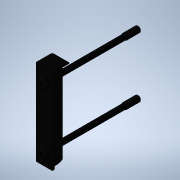
# Autodesk Inventor part: 8092760 MS4-MV-B---(46_high_m)
Saved by Autodesk Inventor 2024.3 (Build 283343000, 343)
## iProperties
Category: PARTsolutions
Company: FESTO
Created: 2025-04-26
Part Number: 8092760 MS4-MV-B---(46_high_m)
Material: Generic
Catalog Web Link: www.cadenas.de
Description: MS4-MV-B_m-module connector
Vendor: FESTO
Document SubType Name: Modeling
Designer: psAdmin
Manufacturer: FESTO
Mass: 2.10543 g
Surface Area: 22.3124 cm^2
Volume: 2.10543 cm^3
Density: 1 g/cm^3
Appearance: PSOLRGB-175-175-175
PSOL_IDENT_0: {$CADENAS_DATA/23d-libs/festo/parts/m/ms4/parts/zubehoer/ms4_mv_b.prj},223 {VTYP=3D},{NB=8092760 MS4
PSOL_IDENT_1: -MV-B---(46_high_m)},{LINA=8092760 MS4-MV-B---(46_high_m)},{NN=MS4-MV-B_m},{DATE=08.04.2024 08:15:04
PSOL_IDENT_2: },{GEOMDATE=08.04.2024 08:15:00},{VERSION=},{LINEID=10},{WBVAR=LODLEVEL,SCREW},{WBNUMERIC=SCREW}  {N
PSOL_IDENT_3: B=8092760 MS4-MV-B---(46_high_m)},{LINA=8092760 MS4-MV-B---(46_high_m)},{KT=DUMMY},{TNR=8092760},{TY
PSOL_IDENT_4: P=MS4-MV-B},{VER=1},{LODDEST=mechanical},{LODLEVEL=high},{LODLEVELX='high', 'High', 'medium', 'Mediu
PSOL_IDENT_5: m','low','Low'},{SCREW=46.0},{SCREW1=42.7,46},{X1=6.600}
NB: 8092760 MS4-MV-B---(46_high_m)
NN: MS4-MV-B_m
NT: module connector
NBSYN: $TNR. $TYP.---($SCREW._$LODLEVEL._m)
LINA: 8092760 MS4-MV-B---(46_high_m)
CATALOG: Festo
TNR: 8092760
TYP: MS4-MV-B
VER: 1
LODLEVEL: High
SCREW: 46
X1: 6.6
SUPPLIER: FESTO
ARTICLENO: 8092760 MS4-MV-B---(46_high_m)
BOMINFO: 8092760 MS4-MV-B---(46_high_m)
CREATOR: CADENAS GmbH
Title: 8092760 MS4-MV-B---(46_high_m)
Author: Cadenas PARTsolutions
Comments: module connector
Autodesk Inventor part; units mm, degrees
sketch "Sketch_1" plane through (0, 0, 0) normal (1, 0, 0) x (0, 1, 0)
  line L0 (22, 5.4) -> (-20.8, 5.4)
  arc A0 (-20.8, 5.4) -> (-21, 5.2) centre (-20.8, 5.2) ccw
  line L1 (-21, 5.2) -> (-21, 1.1788)
  arc A1 (-21, 1.1788) -> (-20.9463, 1.0424) centre (-20.8, 1.1788) ccw
  line L2 (-20.9463, 1.0424) -> (-20.419, 0.477)
  arc A2 (-20.419, 0.477) -> (-19.322, 0) centre (-19.322, 1.5) ccw
  line L3 (-19.322, 0) -> (21.2, 0)
  line L4 (21.2, 0) -> (21.2, -3.3)
  line L5 (21.2, -3.3) -> (21.6171, -3.3)
  line L6 (21.6171, -3.3) -> (22.1063, -2.2509)
  arc A3 (22.1063, -2.2509) -> (22.2, -1.8283) centre (21.2, -1.8283) ccw
  line L7 (22.2, -1.8283) -> (22.2, 5.2)
  arc A4 (22.2, 5.2) -> (22, 5.4) centre (22, 5.2) ccw
  constraints: 16 end point, 10 point on circle, 5 centre point
extrude "Extrusion1" add sketch "Sketch_1" along normal mid plane 8
sketch "Sketch_2" plane through (0, 0, 0) normal (1, 0, 0) x (0, 1, 0)
  line L0 (15, 4.2) -> (15, 5.4)
  line L1 (15, 5.4) -> (18.05, 5.4)
  line L2 (18.05, 5.4) -> (18.05, 4.2)
  line L3 (18.05, 4.2) -> (15, 4.2)
  line L4 (15, 4.2) -> (15, 5.4)
  constraints: 10 end point
revolve "Revolution1" cut sketch "Sketch_2" angle 360 about axis through (0, 15, 4.2) along (0, 0, -1)
sketch "Sketch_3" plane through (0, 0, 0) normal (1, 0, 0) x (0, 1, 0)
  line L0 (-15, 4.2) -> (-15, 5.4)
  line L1 (-15, 5.4) -> (-11.95, 5.4)
  line L2 (-11.95, 5.4) -> (-11.95, 4.2)
  line L3 (-11.95, 4.2) -> (-15, 4.2)
  line L4 (-15, 4.2) -> (-15, 5.4)
  constraints: 10 end point
revolve "Revolution2" cut sketch "Sketch_3" angle 360 about axis through (0, -15, 4.2) along (0, 0, -1)
sketch "Sketch_6" plane through (0, -21.6, 0) normal (0, 1, 0) x (1, 0, 0)
  arc A0 (-1.7301, -0.5774) -> (-2.6364, 0) centre (-2.6364, -1) ccw
  line L0 (-1.7301, -0.5774) -> (-1.2427, -1.6226)
  arc A1 (-1.2427, -1.6226) -> (-0.3364, -2.2) centre (-0.3364, -1.2) ccw
  line L1 (-0.3364, -2.2) -> (0.3364, -2.2)
  arc A2 (0.3364, -2.2) -> (1.2427, -1.6226) centre (0.3364, -1.2) ccw
  line L2 (1.2427, -1.6226) -> (1.7301, -0.5774)
  arc A3 (2.6364, 0) -> (1.7301, -0.5774) centre (2.6364, -1) ccw
  line L3 (2.6364, 0) -> (-2.6364, 0)
  constraints: 8 end point, 8 point on circle, 4 centre point
extrude "Extrusion2" cut sketch "Sketch_6" along normal blind 42.8
sketch "Sketch_4" plane through (0, 0, 0) normal (1, 0, 0) x (0, 1, 0)
  line L0 (15, -41.8) -> (15, 6.6)
  line L1 (15, 6.6) -> (16.6, 6.6)
  line L2 (16.6, 6.6) -> (17.471, 6.283)
  arc A0 (17.8, 5.8131) -> (17.471, 6.283) centre (17.3, 5.8131) ccw
  line L3 (17.8, 5.8131) -> (17.8, 4.2)
  line L4 (17.8, 4.2) -> (16.275, 4.2)
  line L5 (16.275, 4.2) -> (16.275, -34.575)
  line L6 (16.275, -34.575) -> (16.5, -34.8)
  line L7 (16.5, -34.8) -> (16.5, -41.4935)
  line L8 (16.5, -41.4935) -> (16.1935, -41.8)
  line L9 (16.1935, -41.8) -> (15, -41.8)
  line L10 (15, -41.8) -> (15, 6.6)
  constraints: 22 end point, 2 point on circle, 1 centre point
revolve "Revolution3" add sketch "Sketch_4" angle 360 about axis through (0, 15, -41.8) along (0, 0, -1)
thread "Thread1" size "M3x0.5" class "6g" standard "ISO Metric profile" full length
sketch "Sketch_5" plane through (0, 0, 0) normal (1, 0, 0) x (0, 1, 0)
  line L0 (-15, -41.8) -> (-15, 6.6)
  line L1 (-15, 6.6) -> (-13.4, 6.6)
  line L2 (-13.4, 6.6) -> (-12.529, 6.283)
  arc A0 (-12.2, 5.8131) -> (-12.529, 6.283) centre (-12.7, 5.8131) ccw
  line L3 (-12.2, 5.8131) -> (-12.2, 4.2)
  line L4 (-12.2, 4.2) -> (-13.725, 4.2)
  line L5 (-13.725, 4.2) -> (-13.725, -34.575)
  line L6 (-13.725, -34.575) -> (-13.5, -34.8)
  line L7 (-13.5, -34.8) -> (-13.5, -41.4935)
  line L8 (-13.5, -41.4935) -> (-13.8065, -41.8)
  line L9 (-13.8065, -41.8) -> (-15, -41.8)
  line L10 (-15, -41.8) -> (-15, 6.6)
  constraints: 22 end point, 2 point on circle, 1 centre point
revolve "Revolution4" add sketch "Sketch_5" angle 360 about axis through (0, -15, -41.8) along (0, 0, -1)
thread "Thread2" size "M3x0.5" class "6g" standard "ISO Metric profile" full length
sketch "Sketch_7" plane through (0, 15, 6.6) normal (0, 0, 1) x (0, 1, 0)
  line L0 (-1, -0.5774) -> (0, -1.1547)
  line L1 (0, -1.1547) -> (1, -0.5774)
  line L2 (1, -0.5774) -> (1, 0.5774)
  line L3 (1, 0.5774) -> (0, 1.1547)
  line L4 (0, 1.1547) -> (-1, 0.5774)
  line L5 (-1, 0.5774) -> (-1, -0.5774)
  constraints: 12 end point
extrude "Extrusion3" cut sketch "Sketch_7" against normal blind 1.04
sketch "Sketch_8" plane through (0, -15, 6.6) normal (0, 0, 1) x (0, 1, 0)
  line L0 (-1, -0.5774) -> (0, -1.1547)
  line L1 (0, -1.1547) -> (1, -0.5774)
  line L2 (1, -0.5774) -> (1, 0.5774)
  line L3 (1, 0.5774) -> (0, 1.1547)
  line L4 (0, 1.1547) -> (-1, 0.5774)
  line L5 (-1, 0.5774) -> (-1, -0.5774)
  constraints: 12 end point
extrude "Extrusion4" cut sketch "Sketch_8" against normal blind 1.04
sketch "Sketch_9" plane through (0, 0, 0) normal (0, 0, 1) x (1, 0, 0)
  line L0 (-5, -18.3964) -> (-5, -23.2)
  line L1 (-5, -23.2) -> (5, -23.2)
  line L2 (5, -23.2) -> (5, -18.3964)
  line L3 (5, -18.3964) -> (4, -18.3964)
  arc A0 (3.9732, -18.4964) -> (4, -18.3964) centre (3.8, -18.3964) ccw
  line L4 (3.9732, -18.4964) -> (1.8927, -22.1)
  arc A1 (1.7195, -22.2) -> (1.8927, -22.1) centre (1.7195, -22) ccw
  line L5 (1.7195, -22.2) -> (-1.7195, -22.2)
  arc A2 (-1.8927, -22.1) -> (-1.7195, -22.2) centre (-1.7195, -22) ccw
  line L6 (-1.8927, -22.1) -> (-3.9732, -18.4964)
  arc A3 (-4, -18.3964) -> (-3.9732, -18.4964) centre (-3.8, -18.3964) ccw
  line L7 (-4, -18.3964) -> (-5, -18.3964)
  constraints: 16 end point, 8 point on circle, 4 centre point
extrude "Extrusion5" cut sketch "Sketch_9" along normal blind 4
ref_plane "ANBAU_XY" through (0, 0, -15.2) normal (0, -1, 0) x (1, 0, 0)
ref_plane "ANBAU_YZ" through (0, 0, -15.2) normal (1, 0, 0) x (0, 0, 1)
ref_plane "ANBAU_ZX" through (0, 0, -15.2) normal (0, 0, 1) x (0, -1, 0)
ref_plane "ANBAU_2_XY" through (0, 0, -15.2) normal (1, 0, 0) x (0, 0, -1)
ref_plane "ANBAU_2_YZ" through (0, 0, -15.2) normal (0, 0, -1) x (0, 1, 0)
ref_plane "ANBAU_2_ZX" through (0, 0, -15.2) normal (0, 1, 0) x (1, 0, 0)
ref_plane "IP_ANBAU_XY" through (0, 0, 0) normal (0, 0, -1) x (1, 0, 0)
ref_plane "IP_ANBAU_YZ" through (0, 0, 0) normal (1, 0, 0) x (0, -1, 0)
ref_plane "IP_ANBAU_ZX" through (0, 0, 0) normal (0, -1, 0) x (0, 0, -1)
ref_plane "IP_ANBAU_2_XY" through (0, 0, -15.2) normal (1, 0, 0) x (0, 0, -1)
ref_plane "IP_ANBAU_2_YZ" through (0, 0, -15.2) normal (0, 0, -1) x (0, 1, 0)
ref_plane "IP_ANBAU_2_ZX" through (0, 0, -15.2) normal (0, 1, 0) x (1, 0, 0)
body "Solid1"
